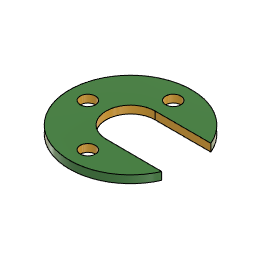
Ex 1 v2 (Autodesk Fusion 360 design; units mm, degrees)
Autodesk Fusion 360 part; units mm, degrees
sketch "Sketch1" plane through (0, 0, 0) normal (0, 0, 1) x (1, 0, 0)
  circle A0 centre (-28, 0) radius 5
  circle A1 centre (0, 28) radius 5
  circle A2 centre (0, -28) radius 5
  line L0 (-0.0776, 15.9998) -> (36.6607, 15.9998)
  line L1 (-0.0776, -15.9998) -> (36.5825, -16.1777)
  arc A3 (36.6607, 15.9998) -> (36.5825, -16.1777) centre (0, 0) ccw
  arc A4 (0.0776, 15.9998) -> (-0.0776, -15.9998) centre (0, 0) ccw
  dimension "d1" = 80
  dimension "d3" = 28
  dimension "d4" = 10
  dimension "d5" = 28
  dimension "d6" = 28
  dimension "d7" = 10
  dimension "d8" = 10
  constraint coincident A3.centre A4.centre
  constraint coincident L0.start A4
  constraint horizontal L0
  constraint tangent L1 A4
  constraint coincident L0 A4.start
  measures "d1" diameter of A3
  measures "d3" distance of A3.centre A0.centre
  measures "d4" diameter of A0
  measures "d5" distance of A3.centre A1.centre
  measures "d6" distance of A3.centre A2.centre
  measures "d7" diameter of A1
  measures "d8" diameter of A2
extrude "Extrude1" add sketch "Sketch1" along normal blind 5
